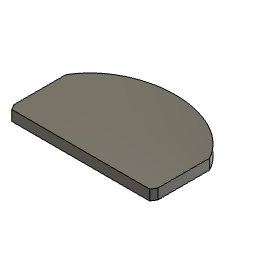
BottomCasePanel v3 (Autodesk Fusion 360 design; units mm, degrees)
Autodesk Fusion 360 part; units mm, degrees
sketch "Sketch1" plane through (0, 0, 0) normal (0, 1, 0) x (1, 0, 0)
  line L0 (-105, -37.7273) -> (-105, 37.7273)
  line L1 (-95, 52.1277) -> (-95, -52.1277)
  line L2 (0, 0) -> (105, 0) construction
  line L3 (0, -20) -> (0, -2.5) construction
  line L4 (0, 92.5) -> (0, 82.5) construction
  ellipse E0 centre (0, 0) end of major axis (-115, 0) minor radius 92.5
  line L5 (115, 0) -> (-115, 0) construction
  line L6 (0, 92.5) -> (0, -92.5) construction
  ellipse E1 centre (0, 0) end of major axis (-105, 0) minor radius 82.5
  line L7 (105, 0) -> (115, 0) construction
  line L8 (0, -1.75) -> (0, -22.5)
  line L9 (95, 52.1277) -> (95, -52.1277)
  line L10 (105, -37.7273) -> (105, 37.7273)
  line L11 (-95, -35.1382) -> (95, -35.1382)
  line L12 (-100.3783, -45.1382) -> (100.3783, -45.1382)
  dimension "d1" = 10
  dimension "d3" = 10
  dimension "d4" = 10
  dimension "d5" = 82.5
  dimension "d7" = 95
  dimension "d13" = 10
  constraint coincident L5.start E0
  constraint coincident L5.end E0
  constraint coincident L4.start E0
  constraint coincident L6.end E0
  constraint coincident L2.start E0.centre
  constraint horizontal L5
  constraint coincident L0.start E0
  constraint coincident L0.end E0
  constraint perpendicular L0 L5
  constraint coincident L1.start E0
  constraint coincident L1.end E0
  constraint perpendicular L1 L5
  constraint tangent L0 E1
  constraint coincident L2.end E1
  constraint coincident L2.end L5
  constraint coincident L4.end E1
  constraint coincident L4.end L6
  constraint symmetric L1.start L8 L9.start
  constraint symmetric L0.end L8 L10.end
  constraint symmetric L0.start L8 L10.start
  constraint symmetric L1.end L8 L9.end
  constraint coincident E1 L11.start
  constraint coincident L1 L11.start
  constraint coincident E1 L11.end
  constraint coincident L9 L11.end
  constraint perpendicular L9 L11
  constraint coincident E0 L12.start
  constraint coincident E0 L12.end
  constraint perpendicular L6 L12
  measures "d1" distance of L0 L1
  measures "d3" distance of L4.start L4.end
  measures "d4" distance of L2.end L5.start
  measures "d5" distance of L2.start L4.end
  measures "d7" distance of L1 L6
  measures "d13" distance of L11 L12
extrude "Extrude1" add sketch "Sketch1" along normal blind 15 contours L0 L1 E0 E1 L12 | L1 E1 | L0 L1 E0 E1 | L1 E1 L12 | E1 L11 L12 | L1 E1 L9 L11 | L1 E0 E1 L9 | E1 L9 L12 | E1 L9 | E0 E1 L9 L10 L12 | E0 E1 L9 L10
equation "d1 = SideWidth"
equation "d3 = SideWidth"
equation "d4 = SideWidth"
equation "d5 = CaseWidth / 2"
equation "SideWidth = 10 mm"
equation "d7 = CaseLength / 2"
equation "CaseLength = 190 mm"
equation "CaseWidth = 165 mm"
equation "PanelHeight = 15 mm"
equation "d11 = PanelHeight"
equation "d13 = SideWidth"
